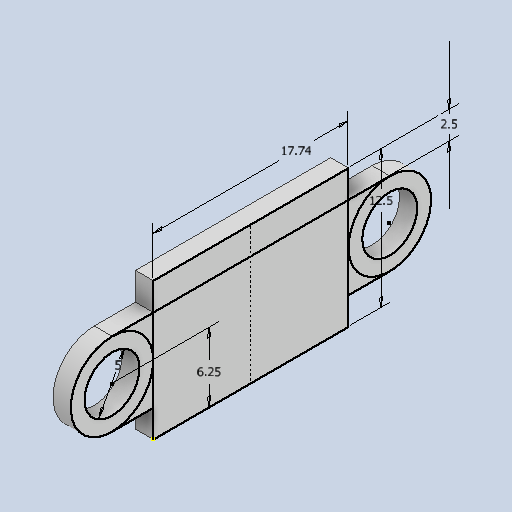
# Autodesk Inventor part: VL53L1X board
Saved by Autodesk Inventor 2022 (Build 260153070, 153G)
## iProperties
Created: 2021-10-27
Part Number: VL53L1X board
Material: Generic
Document SubType Name: Modeling
Designer: a laptop
Density: 1 g/cm^3
Appearance: Default
Author: a laptop
Autodesk Inventor part; units mm, degrees
ref_plane "YZ Plane" through (0, 0, 0) normal (1, 0, 0) x (0, 1, 0)
ref_plane "XZ Plane" through (0, 0, 0) normal (0, 1, 0) x (-1, 0, 0)
ref_plane "XY Plane" through (0, 0, 0) normal (0, 0, 1) x (1, 0, 0)
sketch "Sketch1" plane through (0, 0, 0) normal (1, 0, 0) x (0, 1, 0)
  line L0 (12.5, 0) -> (0, 0)
  line L1 (0, 0) -> (0, -17.74)
  line L2 (0, -17.74) -> (12.5, -17.74)
  line L3 (12.5, -17.74) -> (12.5, 0)
  circle A0 centre (6.25, 3.75) radius 2.5
  line L4 (10, 0) -> (10, -17.74)
  circle A1 centre (6.25, 3.75) radius 3.75
  line L5 (10, 3.75) -> (10, 0)
  line L6 (2.5, 3.75) -> (2.5, 0)
  line L7 (12.5, -8.87) -> (0, -8.87) construction
  circle A2 centre (6.25, -21.49) radius 2.5
  circle A3 centre (6.25, -21.49) radius 3.75
  line L8 (10, -21.49) -> (10, -17.74)
  line L9 (2.5, -21.49) -> (2.5, -17.74)
  dimension "d0" = 17.74
  dimension "d1" = 12.5
  dimension "d2" = 6.25
  dimension "d3" = 5
  dimension "d4" = 2.5
  constraints: 20 end point, 5 symmetric about line, 4 centre point, 4 point on circle, 3 coincident, 3 perpendicular, 3 point on line, 3 tangent, 2 midpoint, 2 parallel, 1 horizontal, 1 vertical, 2 other
  measures "d0" distance of L2.end L0.start
  measures "d1" distance of L1.end L2.end
  measures "d2" horizontal distance of point (0, 0) A0.centre
  measures "d3" diameter of A0
  measures "d4" distance between parallel lines of L3 L4
extrude "Extrusion1" add sketch "Sketch1" against normal blind 1.57
body "Solid1"
